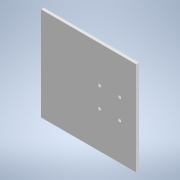
# Autodesk Inventor part: Part5
Saved by Autodesk Inventor 2020.2 (Build 242310000, 310)
## iProperties
Created: 2022-11-01
Part Number: Part5
Material: 一般
Document SubType Name: Modeling
Designer: Administrator
Density: 1 g/cm^3
Appearance: 既定
Author: Administrator
Autodesk Inventor part; units mm, degrees
ref_plane "YZ Plane" through (0, 0, 0) normal (1, 0, 0) x (0, 1, 0)
ref_plane "XZ Plane" through (0, 0, 0) normal (0, 1, 0) x (-1, 0, 0)
ref_plane "XY Plane" through (0, 0, 0) normal (0, 0, 1) x (1, 0, 0)
sketch "スケッチ1" plane through (0, 0, 0) normal (0, 0, 1) x (1, 0, 0)
  circle A0 centre (10.6066, -10.6066) radius 1.5 projected
  circle A1 centre (-10.6066, -10.6066) radius 1.5 projected
  circle A2 centre (10.6066, 10.6066) radius 1.5 projected
  circle A3 centre (-10.6066, 10.6066) radius 1.5 projected
  circle A4 centre (0, 0) radius 6.3 projected
  circle A5 centre (0, 0) radius 19.7 projected
  line L0 (28.0076, -49.2975) -> (-28.0076, -49.2975)
  line L1 (-28.0076, -49.2975) -> (-28.0076, 49.2975)
  line L2 (-28.0076, 49.2975) -> (28.0076, 49.2975)
  line L3 (28.0076, 49.2975) -> (28.0076, -49.2975)
  line L4 (28.0076, -49.2975) -> (-28.0076, 49.2975) construction
  line L5 (-28.0076, -49.2975) -> (28.0076, 49.2975) construction
  line L6 (-28.0076, 49.2975) -> (-72.211, 49.2975)
  line L7 (-72.211, 49.2975) -> (-72.211, -49.3007)
  line L8 (-72.211, -49.3007) -> (-28.0076, -49.3007)
  line L9 (-28.0076, -49.3007) -> (-28.0076, 49.2975)
  point P0 (0, 0)
  point P1 (-28.0076, -6.8711)
  constraints: 20 end point, 4 parallel, 2 horizontal, 2 midpoint, 2 perpendicular
extrude "押し出し1" add sketch "スケッチ1" along normal blind 9.4591 contours A4 | A5 | L0 L1 L2 L3 | L9 L8 L7 L6 L1
